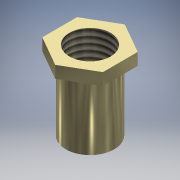
# Autodesk Inventor part: huelse_M3
Saved by Autodesk Inventor 2017 (Build 210142000, 142)
## iProperties
Part Number: huelse_M3
Material: Generisch
Document SubType Name: Modeling
Designer: Philomena-Theresa
Density: 1 g/cm^3
Appearance: Vorgabe
Author: Philomena-Theresa
Autodesk Inventor part; units mm, degrees
ref_plane "YZ Plane" through (0, 0, 0) normal (1, 0, 0) x (0, 1, 0)
ref_plane "XZ Plane" through (0, 0, 0) normal (0, 1, 0) x (-1, 0, 0)
ref_plane "XY Plane" through (0, 0, 0) normal (0, 0, 1) x (1, 0, 0)
sketch "Skizze4" plane through (0, 0, 0) normal (0, 0, 1) x (1, 0, 0)
  line L0 (2.5046, -1.4353) -> (0.0093, -2.8867)
  line L1 (0.0093, -2.8867) -> (-2.4953, -1.4514)
  line L2 (-2.4953, -1.4514) -> (-2.5046, 1.4353)
  line L3 (-2.5046, 1.4353) -> (-0.0093, 2.8867)
  line L4 (-0.0093, 2.8867) -> (2.4953, 1.4514)
  line L5 (2.4953, 1.4514) -> (2.5046, -1.4353)
  point P0 (0, 0)
  point P1 (0, 0)
  dimension "d21" = 5
  constraints: 12 end point, 1 coincident, 13 other
  measures "d21" distance between parallel lines of L4 L1
extrude "Extrusion1" add sketch "Skizze4" along normal blind 1
sketch "Skizze5" plane through (0, 0, 0) normal (0, 0, -1) x (-1, 0, 0)
  circle A0 centre (0, 0) radius 2
  dimension "d7" = 4
  constraints: 1 centre point, 1 coincident
  measures "d7" diameter of A0
extrude "Extrusion2" add sketch "Skizze5" along normal blind 5.5
sketch "Skizze6" plane through (0, 0, 1) normal (0, 0, 1) x (1, 0, 0)
  point P0 (0, 0)
hole "Bohrung1" at (0, 0, 1) direction (0, 0, -1) diameter 3.4 depth 10.65 tip angle 118 clearance for "Flachkopfmaschinenschraube" size "M3" standard "ANSI Metrisches M Profil"
thread "Gewinde2" size "M3x0.5" class "6H" standard "ANSI Metric M Profile" full length
